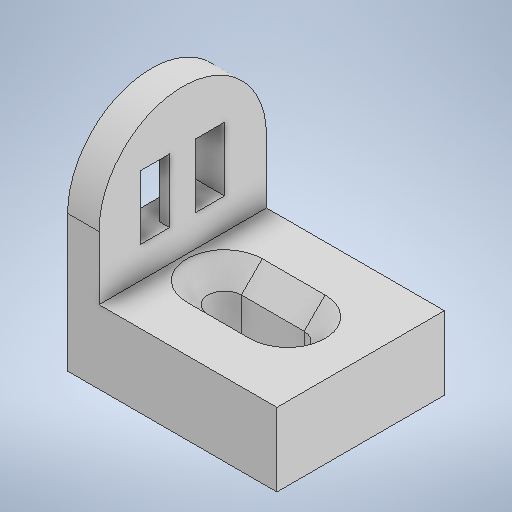
# Autodesk Inventor part: button_mount
Saved by Autodesk Inventor 2025 (Build 290162000, 162)
## iProperties
Created: 2026-04-07
Part Number: button_mount
Material: Generic
Document SubType Name: Modeling
Designer: Luca
Density: 1 g/cm^3
Appearance: Default
Author: Luca
Autodesk Inventor part; units mm, degrees
ref_plane "YZ Plane" through (0, 0, 0) normal (1, 0, 0) x (0, 1, 0)
ref_plane "XZ Plane" through (0, 0, 0) normal (0, 1, 0) x (-1, 0, 0)
ref_plane "XY Plane" through (0, 0, 0) normal (0, 0, 1) x (1, 0, 0)
derived "sk_reservoir.ipt"
sketch "button_mount" plane through (0, -57.9, 0) normal (0, 1, 0) x (-1, 0, 0)
  line L0 (80, 133.17) -> (80, -125.8542)
  line L1 (77.5, -148.4939) -> (77.5, 153.4424)
  line L2 (74.2, -8) -> (54.2, -8)
  line L3 (54.2, -8) -> (54.2, 8)
  line L4 (54.2, 8) -> (74.2, 8)
  line L5 (74.2, 8) -> (74.2, -8)
  circle A0 centre (61.2, 0) radius 1.6 construction
  line L6 (77.2, -8.25) -> (51.2, -8.25)
  line L7 (51.2, -8.25) -> (51.2, 8.25)
  line L8 (51.2, 8.25) -> (77.2, 8.25)
  line L9 (77.2, 8.25) -> (77.2, -8.25)
  circle A1 centre (64.2, 0) radius 1.6
  arc A2 (61.2, 1.6) -> (61.2, -1.6) centre (61.2, 0) ccw
  circle A3 centre (67.2, 0) radius 1.6 construction
  line L10 (61.2, -1.6) -> (67.2, -1.6)
  line L11 (61.2, 1.6) -> (67.2, 1.6)
  arc A4 (67.2, -1.6) -> (67.2, 1.6) centre (67.2, 0) ccw
  line L12 (60.8, 0) -> (62.5, 2.9445)
  line L13 (62.5, 2.9445) -> (65.9, 2.9445)
  line L14 (65.9, 2.9445) -> (67.6, 0)
  line L15 (67.6, 0) -> (65.9, -2.9445)
  line L16 (65.9, -2.9445) -> (62.5, -2.9445)
  line L17 (62.5, -2.9445) -> (60.8, 0)
  point P0 (0, 0)
  point P1 (80, -8)
  point P2 (80, -8)
  point P3 (80, -8)
  point P4 (80, 8)
  point P5 (80, 8)
  point P6 (80, 8)
  point P7 (54.2, 0)
sketch "button" plane through (-80, 0, 0) normal (1, 0, 0) x (0, 1, 0)
  line L0 (-57.9, 133.17) -> (-57.9, -125.8542)
  line L1 (-43.8, -4) -> (-49.9, -4)
  line L2 (-49.9, -4) -> (-49.9, 4)
  line L3 (-49.9, 4) -> (-43.8, 4)
  line L4 (-43.8, 4) -> (-43.8, -4)
  line L5 (-43.8, -1.25) -> (-49.9, -1.25)
  line L6 (-49.9, -1.25) -> (-49.9, 1.25)
  line L7 (-49.9, 1.25) -> (-43.8, 1.25)
  line L8 (-43.8, 1.25) -> (-43.8, -1.25)
  line L9 (-49.9, 0) -> (-0.1295, 0) construction
  line L10 (-132, 0) -> (302, 0) construction
  circle A0 centre (-46.85, 0) radius 6.5
  circle A1 centre (-46.85, 0) radius 6.25
  circle A2 centre (-46.85, 0) radius 5.25
  circle A3 centre (-46.85, 0) radius 5
  circle A4 centre (-46.85, 0) radius 8
  line L11 (-46.85, -8) -> (-57.9, -8)
  line L12 (-46.85, 8) -> (-57.9, 8)
  point P0 (0, 0)
  point P1 (-46.85, 4)
  point P2 (-43.8, 1.25)
extrude "Extrusion1" add sketch "button_mount" along normal blind 5 contours L2 L3 L4 L5 | A1 | A1 L11 L14 L15 L10 | A1 L10 L17 L12 L11 | L11 L12 L13 L14 | L10 L15 L16 L17 | L12 L17 L10 A2 L11 | L11 A4 L10 L15 L14
extrude "Extrusion5" add sketch "button_mount" against normal blind 2 contours L2 L3 L4 L5 | L11 L12 L13 L14 | L10 L15 L16 L17
extrude "Extrusion2" cut sketch "button_mount" along normal through all contours A1 | A1 L11 L14 L15 L10 | A1 L10 L17 L12 L11 | L12 L17 L10 A2 L11 | L11 A4 L10 L15 L14
chamfer "Chamfer1" distance 2 angle 45 4 edges at (-64.2, -52.9, -1.6) (-59.6, -52.9, 0) (-64.2, -52.9, 1.6) (-68.8, -52.9, 0)
extrude "Extrusion3" add sketch "button" against normal blind 3 from surface at 8.8 contours L12 A4 L11 L0 | A4 | A3 L1 | L4 A3 | A3 L2 | L3 A3 | A0 | A1 | A2
extrude "Extrusion4" add sketch "button" against normal blind 1 from surface at 8.8 contours L12 A4 L11 L0 | A4 | A3 L1 | L4 A3 | L5 L2 L7 L4 | A3 L2 | L3 A3 | A0 | A1 | A2
ref_plane "Work Plane21" through (-71.2, 0, 0) normal (1, 0, 0) x (0, 1, 0)
body "Solid1"
